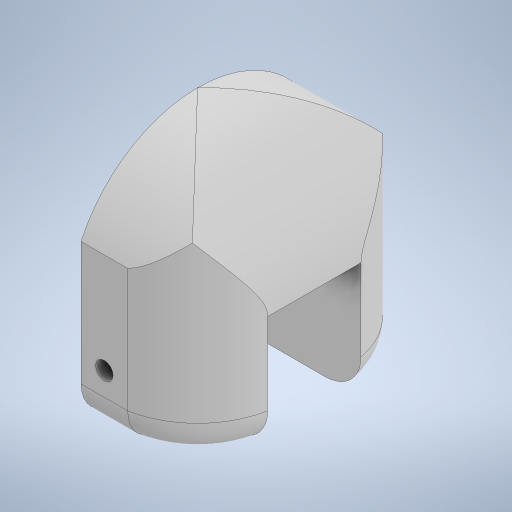
# Autodesk Inventor part: opuszek
Saved by Autodesk Inventor 2024.2 (Build 282272000, 272)
## iProperties
Created: 2024-01-13
Part Number: opuszek
Material: PLA
Document SubType Name: Modeling
Designer: Konrad
Density: 1 g/cm^3
Appearance: Domyślna
Author: Konrad
Autodesk Inventor part; units mm, degrees
ref_plane "YZ Plane" through (0, 0, 0) normal (1, 0, 0) x (0, 1, 0)
ref_plane "XZ Plane" through (0, 0, 0) normal (0, 1, 0) x (-1, 0, 0)
ref_plane "XY Plane" through (0, 0, 0) normal (0, 0, 1) x (1, 0, 0)
sketch "Szkic1" plane through (0, 0, 0) normal (1, 0, 0) x (0, 1, 0)
  line L0 (0, 0) -> (13, 0) construction
  arc A0 (6.5826, -10) -> (13, 0) centre (2, 0) ccw
  arc A1 (13, 0) -> (6.5826, 10) centre (2, 0) ccw
  line L1 (6.5826, -10) -> (-7, -10)
  line L2 (-7, -10) -> (-7, -4)
  line L3 (-7, 4) -> (-7, 10)
  line L4 (-7, 10) -> (6.5826, 10)
  line L5 (-7, -4) -> (3, -4)
  line L6 (3, -4) -> (3, 4)
  line L7 (3, 4) -> (-7, 4)
  line L8 (-7, 4) -> (-7, -4)
  dimension "d9" = 13
  dimension "d14" = 11
  dimension "d22" = 10
  dimension "d36" = 8
  dimension "d37" = 10
  dimension "d38" = 20
  dimension "d39" = 4
  constraints: 18 end point, 4 point on circle, 3 horizontal, 3 perpendicular, 2 centre point, 2 parallel, 2 point on line, 2 symmetric about line, 1 coincident, 1 other
  measures "d9" distance of L0.start L0.end
  measures "d14" radius of A0
  measures "d22" distance from line of L0 L3.end
  measures "d36" distance of L7.end L2.end
  measures "d37" distance of L6.end L7.end
  measures "d38" distance from line of L3 L0.end
  measures "d39" vertical distance of L5.end A0.centre
extrude "Wyciągnięcie proste1" add sketch "Szkic1" along normal blind 10 contours L1 L2 L5 L6 L7 L3 L4 A1 A0
sketch "Szkic5" plane through (0, -7, 4) normal (0, -1, 0) x (1, 0, 0)
  line L0 (0, 6) -> (0, 0) projected
  line L1 (0, 0) -> (10, 0) construction
  line L2 (10, 6) -> (10, 0) projected
  line L3 (0, 6) -> (10, 6) projected
  line L4 (0, 0) -> (0, -8) projected
  line L5 (0, -8) -> (10, -8) construction
  line L6 (10, 0) -> (10, -8) projected
  line L7 (0, 0) -> (10, 0) projected
  line L8 (0, -8) -> (0, -14) construction
  line L9 (0, -14) -> (10, -14) projected
  line L10 (10, -8) -> (10, -14) projected
  line L11 (0, -8) -> (10, -8) construction
  arc A0 (10, 0) -> (4, 6) centre (2.6268, -1.3732) ccw
  line L12 (0, -4) -> (10, -4) construction
  line L13 (0, -14) -> (10, -14) projected
  arc A1 (4, -14) -> (10, -8) centre (2.6268, -6.6268) ccw
  point P0 (4, -14)
  point P1 (10, 0)
  dimension "d40" = 7.5
  dimension "d41" = 4
  constraints: 4 point on circle, 2 centre point, 2 end point, 2 point on line, 1 equal radius, 1 midpoint, 1 other
  measures "d40" radius of A0
  measures "d41" distance of L0.start A0.end
extrude "Wyciągnięcie proste5" cut sketch "Szkic5" against normal through all contours L3 L2 A0 | A1 L10 L9
sketch "Szkic6" plane through (0, -7, -10) normal (0, 0, -1) x (-1, 0, 0)
  line L0 (0, 0) -> (0, 13.5826) projected
  line L1 (0, 0) -> (-4, 0) projected
  line L2 (-10, 0) -> (-4, 0) construction
  line L3 (-10, 10) -> (-10, 0) projected
  line L4 (-10, 10) -> (-10, 19.247) projected
  line L5 (-10, 20) -> (-10, 19.247) projected
  line L6 (0, 20) -> (-10, 20) projected
  line L7 (0, 20) -> (0, 13.5826) projected
  arc A0 (0, 20) -> (-10, 10) centre (0, 10) ccw
  point P0 (0, 7)
  point P1 (-1.9, 19)
  dimension "d44" = 10
  constraints: 2 point on circle, 1 centre point, 1 tangent
  measures "d44" radius of A0
extrude "Wyciągnięcie proste6" cut sketch "Szkic6" against normal through all
fillet "Zaokrąglenie2" radius 3 4 edges at (7.9301, -7, 7.9301) (2, -7, 10) (7.9301, -7, -7.9301) (2, -7, -10)
sketch "Szkic7" plane through (0, 6.5826, 10) normal (0, 0, 1) x (1, 0, 0)
  line L0 (4, -10.5826) -> (0, -10.5826) projected
  line L1 (4, -10.5826) -> (4, 0) projected
  line L2 (0, 0) -> (4, 0) projected
  line L3 (0, 0) -> (0, -10.5826) projected
  circle A0 centre (2, -8.5826) radius 0.75
  line L4 (0, -13.5826) -> (0, -3.5826) projected
  line L5 (0, -13.5826) -> (6.9121, -13.5826) projected
  line L6 (0, -13.5826) -> (0, -3.5826) projected
  line L7 (0, -3.5826) -> (10, -3.5826) projected
  line L8 (10, -10.5826) -> (10, -3.5826) projected
  point P0 (0, -6.5826)
  dimension "d48" = 1.5
  dimension "d49" = 4
  dimension "d50" = 2
  dimension "d51" = 10
  dimension "d52" = 5
  constraints: 1 centre point, 1 other
  measures "d48" diameter of A0
  measures "d49" distance of L2.start L1.end
  measures "d50" distance from line of L3 A0.centre
  measures "d51" distance between parallel lines of L5 L7
  measures "d52" distance from line of L5 A0.centre
extrude "Wyciągnięcie proste7" cut sketch "Szkic7" against normal up to surface (20 mm away) contours A0
equation "\"d39\" = 0.5 * d36"
